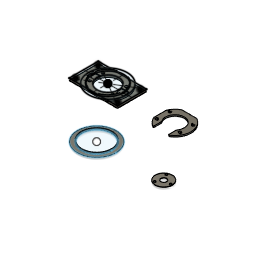
Support ring led Tron v11 (Autodesk Fusion 360 design; units mm, degrees)
Autodesk Fusion 360 part; units mm, degrees
sketch "Esquisse1" plane through (0, 0, 0) normal (0, 1, 0) x (1, 0, 0)
  circle A0 centre (0, 0) radius 35.5
  circle A1 centre (0, 0) radius 34.5
  circle A2 centre (0, 0) radius 24
  circle A3 centre (0, 0) radius 43
  line L0 (-54, -32.5) -> (54, -32.5)
  line L1 (54, -32.5) -> (54, 32.5)
  line L2 (54, 32.5) -> (-54, 32.5)
  line L3 (-54, 32.5) -> (-54, -32.5)
  line L4 (-54, -32.5) -> (54, 32.5) construction
  line L5 (54, -32.5) -> (-54, 32.5) construction
  line L6 (-54, -32.5) -> (-44.8, -32.5) construction
  line L7 (-44.8, -32.5) -> (-44.8, -22.8) construction
  line L8 (-44.8, -22.8) -> (-54, -22.8) construction
  circle A4 centre (-47.05, -25.05) radius 2.25
  line L9 (-54, 0) -> (54, 0) construction
  line L10 (0, 32.5) -> (0, -32.5) construction
  circle A5 centre (-47.05, 25.05) radius 2.25
  circle A6 centre (47.05, 25.05) radius 2.25
  circle A7 centre (47.05, -25.05) radius 2.25
  dimension "d1" = 71
  dimension "d2" = 69
  dimension "d3" = 48
  dimension "d4" = 86
  dimension "d30" = 65
  dimension "d85" = 108
  dimension "d86" = 9.2
  dimension "d87" = 9.7
  dimension "d88" = 2.25
  constraint coincident A0.centre A1.centre
  constraint concentric A0 A2
  constraint concentric A1 A3
  constraint horizontal L0
  constraint perpendicular L0 L1
  constraint parallel L0 L2
  constraint parallel L1 L3
  constraint coincident L4 A0.centre
  constraint coincident L5 A0.centre
  constraint perpendicular L3 L6
  constraint perpendicular L6 L7
  constraint coincident L3 L8.end
  constraint perpendicular L3 L8
  constraint tangent L8 A4
  constraint tangent L7 A4
  constraint midpoint L3 L9.start
  constraint midpoint L1 L9.end
  constraint midpoint L2 L10.start
  constraint midpoint L0 L10.end
  constraint symmetric A4 L9 A5
  constraint symmetric A4 L10 A7
  constraint symmetric L10 A5 A6
  measures "d1" diameter of A0
  measures "d2" diameter of A1
  measures "d3" diameter of A2
  measures "d4" diameter of A3
  measures "d30" distance of L0.end L1.end
  measures "d85" distance of L1 L3
  measures "d86" distance of L0.start L6.end
  measures "d87" distance of L6.end L7.end
  measures "d88" radius of A4
extrude "Extrusion1" add sketch "Esquisse1" against normal blind 5 contours A0 A1 L0 L2 | A0 A3 L0 L2 | A0 A1 L0 L2 | A0 A3 L0 L2 | A1 L0 L2 makes body 1
extrude "Extrusion2" add sketch "Esquisse1" along normal blind 3.2 contours A0 A1 L0 L2 | A0 A1 L0 L2 bodies 1
sketch "Esquisse2" plane through (0, 0, 0) normal (0, 1, 0) x (1, 0, 0)
  line L0 (41, 7) -> (-41, 7)
  line L1 (-41, 7) -> (-41, -7)
  line L2 (-41, -7) -> (41, -7)
  line L3 (41, -7) -> (41, 7)
  line L4 (41, 7) -> (-41, -7) construction
  line L5 (-41, 7) -> (41, -7) construction
  dimension "d9" = 14
  constraint horizontal L0
  constraint perpendicular L0 L1
  constraint parallel L0 L2
  constraint parallel L1 L3
  constraint coincident L4 origin
  constraint coincident L5 origin
  measures "d9" distance of L0.end L1.end
extrude "Extrusion3" cut sketch "Esquisse2" against normal blind 2 bodies 1
extrude "Extrusion4" cut sketch "Esquisse2" along normal blind 4 bodies 1
sketch "Esquisse3" plane through (0, 0, 0) normal (0, 1, 0) x (1, 0, 0)
  line L0 (-49.8557, -7) -> (-35, -7)
  line L1 (-35, -7) -> (-35, 7)
  line L2 (-35, 7) -> (-49.8557, 7)
  line L3 (-49.8557, 7) -> (-49.8557, -7)
  constraint horizontal L0
  constraint vertical L1
  constraint horizontal L2
  constraint vertical L3
extrude "Extrusion5" cut sketch "Esquisse3" against normal blind 5 bodies 1
sketch "Esquisse5" plane through (0, 0, 0) normal (0, 1, 0) x (-1, 0, 0)
  line L0 (22.9565, 7) -> (33.7824, 7)
  arc A0 (33.7824, 7) -> (11.5758, 32.5) centre (0, 0) ccw
  line L1 (-33.7824, 7) -> (-22.9565, 7)
  arc A1 (22.9565, 7) -> (-22.9565, 7) centre (0, 0) ccw
  line L2 (0, 24) -> (0, 30) construction
  line L3 (0, -22.5) -> (0, -28.5) construction
  line L4 (11.5758, 32.5) -> (-11.5758, 32.5)
  arc A2 (-11.5758, 32.5) -> (-33.7824, 7) centre (0, 0) ccw
  line L5 (0, 0) -> (25.9808, -15) construction
  line L6 (0, 0) -> (30, 0) construction
  line L7 (0, 0) -> (25.9808, 15) construction
  line L8 (0, 0) -> (30, 0) construction
  line L9 (0, 0) -> (-25.9808, 15) construction
  line L10 (0, 0) -> (-30, 0) construction
  line L11 (0, 0) -> (-25.9808, -15) construction
  line L12 (0, 0) -> (30, 0) construction
  circle A3 centre (25.9808, -15) radius 1.75
  circle A4 centre (25.9808, -15) radius 3
  circle A5 centre (25.9808, 15) radius 1.75
  circle A6 centre (25.9808, 15) radius 3
  circle A7 centre (-25.9808, -15) radius 1.75
  circle A8 centre (-25.9808, -15) radius 3
  circle A9 centre (-25.9808, 15) radius 1.75
  circle A10 centre (-25.9808, 15) radius 3
  circle A11 centre (-150, 0) radius 30 construction
  line L13 (-150, 0) -> (-124.0192, -15) construction
  line L14 (-150, 0) -> (-120, 0) construction
  line L15 (-150, 0) -> (-124.0192, 15) construction
  line L16 (-150, 0) -> (-120, 0) construction
  line L17 (-150, 0) -> (-175.9808, -15) construction
  line L18 (-150, 0) -> (-120, 0) construction
  line L19 (-150, 0) -> (-175.9808, 15) construction
  line L20 (-150, 0) -> (-120, 0) construction
  circle A12 centre (-124.0192, -15) radius 1.75
  circle A13 centre (-175.9808, -15) radius 1.75
  circle A14 centre (-124.0192, 15) radius 1.75
  circle A15 centre (-175.9808, 15) radius 1.75
  circle A16 centre (-150, 0) radius 21
  circle A17 centre (-150, 0) radius 36
  line L21 (-193, 32) -> (-107, 32)
  line L22 (-107, 32) -> (-107, -32)
  line L23 (-107, -32) -> (-193, -32)
  line L24 (-193, -32) -> (-193, 32)
  line L25 (-193, 32) -> (-107, -32) construction
  line L26 (-107, 32) -> (-193, -32) construction
  line L27 (-166.4924, -32) -> (-133.5076, -32)
  line L28 (-133.5076, -32) -> (-133.5076, 32)
  line L29 (-133.5076, 32) -> (-166.4924, 32)
  line L30 (-166.4924, 32) -> (-166.4924, -32)
  line L31 (-166.4924, -32) -> (-133.5076, 32) construction
  line L32 (-133.5076, -32) -> (-166.4924, 32) construction
  line L33 (-116.7328, -13.7585) -> (-111.2672, -13.7585)
  line L34 (-111.2672, -13.7585) -> (-111.2672, 13.7585)
  line L35 (-111.2672, 13.7585) -> (-116.7328, 13.7585)
  line L36 (-116.7328, 13.7585) -> (-116.7328, -13.7585)
  line L37 (-116.7328, -13.7585) -> (-111.2672, 13.7585) construction
  line L38 (-111.2672, -13.7585) -> (-116.7328, 13.7585) construction
  circle A18 centre (-124.0192, -15) radius 3
  circle A19 centre (-124.0192, 15) radius 3
  circle A20 centre (-175.9808, -15) radius 3
  circle A21 centre (-175.9808, 15) radius 3
  line L39 (-194, 16) -> (-106, 16)
  line L40 (-106, 16) -> (-106, -16)
  line L41 (-106, -16) -> (-194, -16)
  line L42 (-194, -16) -> (-194, 16)
  line L43 (-194, 16) -> (-106, -16) construction
  line L44 (-106, 16) -> (-194, -16) construction
  point P0 (-150, 0)
  point P1 (-150, 0)
  point P2 (-150, 0)
  point P3 (-150, 0)
  point P4 (-114, 0)
  point P5 (-150, 0)
  dimension "d31" = 30
  dimension "d32" = 30
  dimension "d33" = 30
  dimension "d34" = 30
  dimension "d35" = 30
  dimension "d36" = 30
  dimension "d37" = 150
  dimension "d38" = 30
  dimension "d39" = 3.5
  dimension "d40" = 6
  dimension "d41" = 3.5
  dimension "d42" = 6
  dimension "d43" = 3.5
  dimension "d44" = 6
  dimension "d45" = 3.5
  dimension "d46" = 6
  dimension "d51" = 60
  dimension "d52" = 30
  dimension "d54" = 30
  dimension "d56" = 150
  dimension "d58" = 150
  dimension "d60" = 3.5
  dimension "d61" = 3.5
  dimension "d62" = 3.5
  dimension "d63" = 3.5
  dimension "d66" = 42
  dimension "d69" = 72
  dimension "d72" = 86
  dimension "d73" = 64
  dimension "d78" = 6
  dimension "d79" = 6
  dimension "d80" = 6
  dimension "d81" = 6
  dimension "d82" = 32
  constraint midpoint A1 L2.start
  constraint vertical L2
  constraint vertical L3
  constraint horizontal L6
  constraint coincident A0.centre A1.centre
  constraint horizontal L8
  constraint horizontal L10
  constraint horizontal L12
  constraint coincident L5.end A3.centre
  constraint concentric A3 A4
  constraint coincident L7.end A5.centre
  constraint concentric A5 A6
  constraint coincident L11.end A7.centre
  constraint concentric A7 A8
  constraint coincident L9.end A9.centre
  constraint concentric A9 A10
  constraint horizontal L14
  constraint coincident P5 P3
  constraint horizontal L16
  constraint horizontal L18
  constraint horizontal L20
  constraint coincident L13.end A12.centre
  constraint coincident L17.end A13.centre
  constraint coincident L15.end A14.centre
  constraint coincident L19.end A15.centre
  constraint concentric A11 A16
  constraint concentric A16 A17
  constraint horizontal L21
  constraint perpendicular L21 L22
  constraint parallel L21 L23
  constraint parallel L22 L24
  constraint coincident L25 P5
  constraint coincident L26 P5
  constraint horizontal L27
  constraint perpendicular L27 L28
  constraint parallel L27 L29
  constraint parallel L28 L30
  constraint coincident A17 L27.start
  constraint coincident L23 L27.start
  constraint coincident L31 P5
  constraint coincident L32 P5
  constraint horizontal L33
  constraint perpendicular L33 L34
  constraint parallel L33 L35
  constraint parallel L34 L36
  constraint coincident A17 L33.start
  constraint coincident L37 P4
  constraint coincident L38 P4
  constraint coincident A17 P4
  constraint concentric A12 A18
  constraint concentric A14 A19
  constraint concentric A13 A20
  constraint concentric A15 A21
  constraint horizontal L39
  constraint perpendicular L39 L40
  constraint parallel L39 L41
  constraint parallel L40 L42
  constraint coincident L43 P5
  constraint coincident L44 P5
  measures "d31" distance of A0.centre L5.end
  measures "d32" angle of L5 L6
  measures "d33" angle of L7 L8
  measures "d34" distance of A0.centre L7.end
  measures "d35" angle of L9 L10
  measures "d36" distance of A0.centre L9.end
  measures "d37" angle of L11 L12
  measures "d38" distance of A0.centre L11.end
  measures "d39" diameter of A3
  measures "d40" diameter of A4
  measures "d41" diameter of A5
  measures "d42" diameter of A6
  measures "d43" diameter of A7
  measures "d44" diameter of A8
  measures "d45" diameter of A9
  measures "d46" diameter of A10
  measures "d51" diameter of A11
  measures "d52" angle of L13 L14
  measures "d54" angle of L15 L16
  measures "d56" angle of L17 L18
  measures "d58" angle of L19 L20
  measures "d60" diameter of A12
  measures "d61" diameter of A13
  measures "d62" diameter of A14
  measures "d63" diameter of A15
  measures "d66" diameter of A16
  measures "d69" diameter of A17
  measures "d72" distance of L22.end L23.end
  measures "d73" distance of L21.end L22.end
  measures "d78" diameter of A18
  measures "d79" diameter of A19
  measures "d80" diameter of A20
  measures "d81" diameter of A21
  measures "d82" distance of L39.end L40.end
extrude "Extrusion10" cut sketch "Esquisse5" against normal blind 6 contours A3 | A5 | A7 | A9 bodies 1
extrude "Extrusion11" cut sketch "Esquisse5" against normal blind 3 contours A4 | A6 | A8 | A10 bodies 1
extrude "Extrusion12" add sketch "Esquisse5" against normal blind 3 separate body contours A12 A18 L41 | A12 A18 L41 | A16 A17 L28 L36 A18 A19 L39 L41 | A17 L28 A18 L41 | A16 L28 L41 | A16 L23 L27 L28 L30 L41 | A17 L30 A20 L41 | A16 L30 L41 | A16 A17 L30 A20 A21 L39 L41 | A17 L28 A19 L39 | A17 L30 A21 L39 | A13 A20 L41 | A13 A20 L41 | A14 A19 L39 | A14 A19 L39 | A15 A21 L39 | A15 A21 L39 makes body 2
fillet "Congé1" radius 1 2 edges at (133.5076, -1.5, 32) (133.5076, -1.5, 13) on bodies 2
fillet "Congé2" radius 1 2 edges at (166.4924, -1.5, 13) (166.4924, -1.5, 32) on bodies 2
sketch "Esquisse6" plane through (0, 0, 0) normal (0, 1, 0) x (1, 0, 0)
extrude "Extrusion13" add sketch "Esquisse5" along normal blind 1.8 contours A12 A18 L41 | A13 A20 L41 | A14 A19 L39 | A15 A21 L39 picked at (-125.6362, -12.9921) picked at (-177.5977, -12.9921) picked at (-125.6362, 12.9921) picked at (-177.5977, 12.9921) bodies 2
extrude "Extrusion14" add sketch "Esquisse1" against normal blind 5 contours A3 L0 L1 L2 | A3 L0 L2 L3 bodies 1
extrude "Extrusion15" cut sketch "Esquisse1" against normal blind 4 contours A3 L0 L1 L2 | A3 L0 L2 L3 bodies 1
sketch "Esquisse7" plane through (0, 0, 0) normal (0, 1, 0) x (1, 0, 0)
  circle A0 centre (100, -125) radius 43
  circle A1 centre (100, -125) radius 34.25
  circle A2 centre (100, -125) radius 33
  dimension "d93" = 86
  dimension "d94" = 68.5
  dimension "d95" = 66
  constraint concentric A0 A1
  constraint concentric A0 A2
  measures "d93" diameter of A0
  measures "d94" diameter of A1
  measures "d95" diameter of A2
extrude "Extrusion16" add sketch "Esquisse7" along normal blind 3 separate body contours A1 makes body 3
extrude "Extrusion17" add sketch "Esquisse7" along normal blind 0.2 contours A0 bodies 3
sketch "Esquisse8" plane through (0, 0, 0) normal (0, 1, 0) x (1, 0, 0)
  circle A0 centre (250, -125) radius 6.35
  circle A1 centre (250, -125) radius 19.05
  line L0 (250, -125) -> (275, -125) construction
  line L1 (250, -125) -> (238.2201, -104.5966) construction
  line L2 (250, -125) -> (273.5599, -125) construction
  line L3 (250, -125) -> (238.1467, -145.5305) construction
  line L4 (250, -125) -> (273.7065, -125) construction
  line L5 (240.7195, -141.0743) -> (242.4695, -138.0432) construction
  line L6 (240.475, -108.5022) -> (242.225, -111.5333) construction
  line L7 (269.05, -125) -> (265.55, -125) construction
  circle A2 centre (242.225, -111.5333) radius 2.25
  circle A3 centre (265.55, -125) radius 2.25
  circle A4 centre (242.4695, -138.0432) radius 2.25
  dimension "d100" = 12.7
  dimension "d101" = 38.1
  dimension "d102" = 120
  dimension "d103" = 120
  dimension "d104" = 3.5
  dimension "d105" = 3.5
  dimension "d106" = 3.5
  dimension "d107" = 4.5
  dimension "d108" = 4.5
  dimension "d109" = 4.5
  constraint concentric A0 A1
  constraint coincident A0.centre A1.centre
  constraint horizontal L0
  constraint horizontal L2
  constraint horizontal L4
  constraint coincident L3 L5.start
  constraint parallel L3 L5
  constraint coincident L1 L6.start
  constraint coincident A1 L6.start
  constraint parallel L1 L6
  constraint coincident A1 L7.start
  constraint coincident L4 L7.start
  constraint parallel L4 L7
  constraint coincident L6.end A2.centre
  constraint coincident L7.end A3.centre
  constraint coincident L5.end A4.centre
  measures "d100" diameter of A0
  measures "d101" diameter of A1
  measures "d102" angle of L1 L2
  measures "d103" angle of L3 L4
  measures "d104" distance of L5.start L5.end
  measures "d105" distance of L6.start L6.end
  measures "d106" distance of L7.start L7.end
  measures "d107" diameter of A2
  measures "d108" diameter of A3
  measures "d109" diameter of A4
extrude "Extrusion18" add sketch "Esquisse8" along normal blind 1 separate body makes body 4
